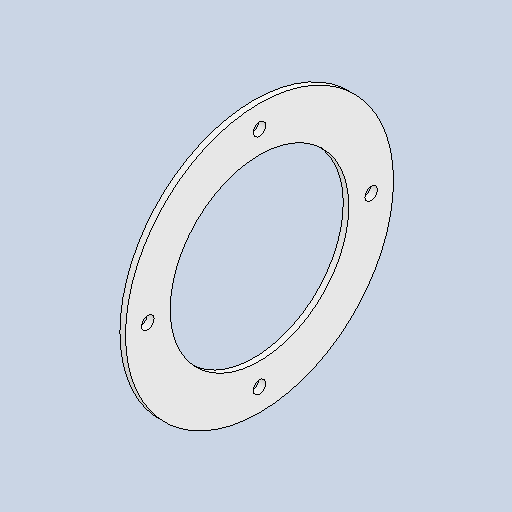
# Autodesk Inventor part: joint3_carrier
Saved by Autodesk Inventor 2025.3 (Build 293356030, 356C)
## iProperties
Created: 2025-11-19
Part Number: joint3_carrier
Material: PLA filament
Document SubType Name: Modeling
Designer: MSI
Mass: 9.66838 g
Surface Area: 90.8549 cm^2
Volume: 8.05698 cm^3
Density: 1.2 g/cm^3
Appearance: 일반
Author: MSI
Autodesk Inventor part; units mm, degrees
ref_plane "YZ Plane" through (0, 0, 0) normal (1, 0, 0) x (0, 1, 0)
ref_plane "XZ Plane" through (0, 0, 0) normal (0, 1, 0) x (-1, 0, 0)
ref_plane "XY Plane" through (0, 0, 0) normal (0, 0, 1) x (1, 0, 0)
sketch "스케치1" plane through (0, 0, 0) normal (1, 0, 0) x (0, 1, 0)
  circle A0 centre (0, 0) radius 40 construction
  circle A1 centre (0, 0) radius 48
  circle A2 centre (0, 0) radius 32
  dimension "d0" = 80
  dimension "d1" = 8
  dimension "d2" = 8
  constraints: 3 centre point, 1 coincident
  measures "d0" diameter of A0
  measures "d1" radial gap between concentric circles of A0 A1
  measures "d2" radial gap between concentric circles of A0 A2
extrude "돌출1" add sketch "스케치1" along normal blind 2
sketch "스케치3" plane through (0, 0, 0) normal (-1, 0, 0) x (0, 0, 1)
  circle A0 centre (0, 40) radius 5
  point P0 (0, 0)
  dimension "d16" = 10
  dimension "d17" = 40
  constraints: 1 centre point, 1 vertical alignment
  measures "d16" diameter of A0
  measures "d17" distance of point (0, 0) A0.centre
extrude "돌출2" add sketch "스케치3" along normal blind 0.5
sketch "스케치2" plane through (2, 0, 0) normal (1, 0, 0) x (0, 0, -1)
  line L0 (0, 0) -> (0, 40)
  dimension "d5" = 40
  constraints: 2 end point, 1 coincident, 1 vertical
  measures "d5" distance of L0.start L0.end
hole "구멍1" at (2, 40, 0) direction (-1, 0, 0) diameter 4.5 end through all clearance for "Countersunk Flat Head Screw ISO 2009/7046" size "M4" standard "ISO"
pattern_circular "원형 패턴1" count 4 over 360 about axis through (0, 0, 0) along (1, 0, 0) of "구멍1", "돌출2"
fillet "모깎기1" radius 1 4 edges at (0, 40, -5) (0, 5, 40) (0, -40, 5) (0, -5, -40)
equation "\"joint4_belt_centor\" = 157.367"
equation "\"joint4_axis2_L\" = 58.803"
equation "\"joint4_axis2_b1\" = 35"
equation "\"joint4_axis2_d\" = 19"
equation "\"joint4_miter_m\" = 2"
equation "\"joint4_miter_a\" = 20deg"
equation "\"joint4_miter_z\" = 79"
equation "\"joint4_miter_b\" = 6.90139"
equation "\"joint4_axis3_L\" = 23.5"
equation "\"joint3_belt_centor\" = 157.367"
equation "\"joint3_axis2_L\" = 71.5"
equation "\"joint3_axis2_b1\" = 38"
equation "\"joint3_axis2_d\" = 29"
equation "\"joint3_planetary_m\" = 2"
equation "\"joint3_planetary_a\" = 20deg"
equation "\"joint3_planetary_np\" = 4"
equation "\"joint3_sun_b\" = 19"
equation "\"joint3_planet_b\" = 19"
equation "\"joint3_ring_b\" = 18"
equation "\"joint3_axis3_d\" = 29"
equation "\"joint3_miter_m\" = 4"
equation "\"joint3_miter_a\" = 20deg"
equation "\"joint3_miter_z1\" = 26"
equation "\"joint3_axis4_L\" = 43.706"
equation "\"joint3_miter_b\" = 25.07657"
equation "\"joint3_miter_z2\" = 39"
